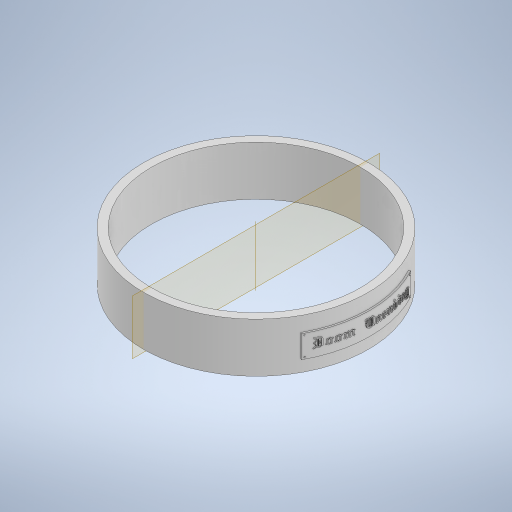
# Autodesk Inventor part: DoomUnending
Saved by Autodesk Inventor 2023 (Build 270158000, 158)
## iProperties
Created: 2023-04-08
Part Number: DoomUnending
Material: Generic
Document SubType Name: Modeling
Designer: dntpa
Density: 1 g/cm^3
Appearance: Default
Author: dntpa
## iProperties of the stored document CanisInvictoria_3DPrint.ipt
Created: 2023-04-08
Part Number: CanisInvictoria_3DPrint
Material: Generic
Document SubType Name: Modeling
Designer: dntpa
Density: 1 g/cm^3
Appearance: Default
Author: dntpa
Autodesk Inventor part; units mm, degrees
ref_plane "XZ Plane" through (0, 0, 0) normal (0, 1, 0) x (-1, 0, 0)
ref_plane "XY Plane" through (0, 0, 0) normal (0, 0, 1) x (1, 0, 0)
sketch "Sketch1" plane through (0, 0, 0) normal (0, 1, 0) x (-1, 0, 0)
  circle A0 centre (0, 0) radius 50
  circle A1 centre (0, 0) radius 46.5
  dimension "d0" = 100
  dimension "d1" = 93
  constraints: 2 centre point, 2 coincident
  measures "d0" diameter of A0
  measures "d1" diameter of A1
extrude "Extrusion1" add sketch "Sketch1" along normal blind 22
ref_plane "Work Plane1" through (60, 0, 0) normal (1, 0, 0) x (0, 1, 0)
sketch "Text" plane through (60, 0, 0) normal (1, 0, 0) x (0, 1, 0)
  line L0 (15.4535, 25) -> (15.4535, -25) construction
  line L1 (15.4535, -25) -> (5.4535, -25) construction
  line L2 (5.4535, -25) -> (5.4535, 25) construction
  line L3 (5.4535, 25) -> (15.4535, 25) construction
  line L4 (22, -50) -> (22, 50) projected
  line L5 (5.4535, 25) -> (15.4535, 25)
  line L6 (15.4535, 25) -> (15.4535, -25)
  line L7 (15.4535, -25) -> (5.4535, -25)
  line L8 (5.4535, -25) -> (5.4535, 25)
  line L9 (15.4535, 25) -> (15.4535, 0)
  line L10 (15.4535, 0) -> (15.4535, -25)
  circle A0 centre (14.7035, 24.25) radius 0.375
  line L11 (22, 0) -> (0, 0)
  line L12 (10.4535, 25) -> (10.4535, -25)
  circle A1 centre (14.7035, -24.25) radius 0.375
  circle A2 centre (6.2035, 24.25) radius 0.375
  circle A3 centre (6.2035, -24.25) radius 0.375
  line L13 (9.6365, 18.3354) -> (9.6365, 18.7286)
  line L14 (9.6365, 18.7286) -> (9.4598, 19.0748)
  line L15 (9.4598, 19.0748) -> (9.0883, 19.45)
  line L16 (9.0883, 19.45) -> (9.2758, 19.8359)
  line L17 (9.2758, 19.8359) -> (9.2758, 20.7232)
  spline S0 degree 2 poles (9.2758, 20.7232) (9.2578, 20.7881) (9.1424, 21.2606) (9.0414, 21.6754) knots 0 0 0 1 2 2 2
  line L18 (9.0414, 21.6754) -> (9.2037, 21.4265)
  line L19 (9.2037, 21.4265) -> (9.5319, 20.9288)
  line L20 (9.5319, 20.9288) -> (9.7195, 20.3733)
  line L21 (9.7195, 20.3733) -> (9.7195, 19.8647)
  line L22 (9.7195, 19.8647) -> (12.5328, 19.8647)
  line L23 (12.5328, 19.8647) -> (12.5328, 20.9179)
  spline S1 degree 2 poles (12.5328, 20.9179) (12.5689, 21.0009) (12.6627, 21.1885) (12.7204, 21.2967) knots 0 0 0 1 2 2 2
  spline S2 degree 2 poles (12.7204, 21.2967) (12.7709, 21.3472) (12.8971, 21.4734) (12.9764, 21.5491) knots 0 0 0 1 2 2 2
  line L24 (12.9764, 21.5491) -> (12.9764, 18.9089)
  line L25 (12.9764, 18.9089) -> (12.7853, 18.5266)
  line L26 (12.7853, 18.5266) -> (12.403, 18.3354)
  line L27 (12.403, 18.3354) -> (9.6365, 18.3354)
  line L28 (9.705, 18.7791) -> (10.5562, 18.7791)
  line L29 (10.5562, 18.7791) -> (10.7222, 19.1073)
  line L30 (10.7222, 19.1073) -> (10.7222, 19.45)
  line L31 (10.7222, 19.45) -> (10.5562, 19.7782)
  line L32 (10.5562, 19.7782) -> (9.7195, 19.7782)
  line L33 (9.7195, 19.7782) -> (9.7195, 19.6339)
  spline S3 degree 2 poles (9.7195, 19.6339) (9.7159, 19.6303) (9.6329, 19.3634) (9.5427, 19.1037) knots 0 0 0 1 2 2 2
  line L34 (9.5427, 19.1037) -> (9.705, 18.7791)
  spline S4 degree 2 poles (10.5743, 20.3228) (10.4949, 20.3589) (10.3074, 20.4491) (10.1956, 20.5068) knots 0 0 0 1 2 2 2
  spline S5 degree 2 poles (10.1956, 20.5068) (10.1451, 20.5573) (10.0224, 20.6871) (9.9431, 20.7665) knots 0 0 0 1 2 2 2
  line L35 (9.9431, 20.7665) -> (10.9061, 20.7665)
  line L36 (10.9061, 20.7665) -> (10.9061, 21.0694)
  line L37 (10.9061, 21.0694) -> (10.6681, 21.3111)
  line L38 (10.6681, 21.3111) -> (11.1406, 21.3111)
  line L39 (11.1406, 21.3111) -> (11.3498, 21.1055)
  line L40 (11.3498, 21.1055) -> (11.3498, 20.7665)
  line L41 (11.3498, 20.7665) -> (11.4976, 20.7665)
  spline S6 degree 2 poles (11.4976, 20.7665) (11.5806, 20.7304) (11.7645, 20.6402) (11.8764, 20.5825) knots 0 0 0 1 2 2 2
  spline S7 degree 2 poles (11.8764, 20.5825) (11.9269, 20.532) (12.0495, 20.4022) (12.1288, 20.3228) knots 0 0 0 1 2 2 2
  line L42 (12.1288, 20.3228) -> (10.5743, 20.3228)
  line L43 (11.696, 18.7791) -> (12.3777, 18.7791)
  line L44 (12.3777, 18.7791) -> (12.5328, 18.9342)
  line L45 (12.5328, 18.9342) -> (12.5328, 19.7782)
  line L46 (12.5328, 19.7782) -> (11.696, 19.7782)
  line L47 (11.696, 19.7782) -> (11.5301, 19.4463)
  line L48 (11.5301, 19.4463) -> (11.5301, 19.1073)
  line L49 (11.5301, 19.1073) -> (11.696, 18.7791)
  line L50 (10.65, 18.7791) -> (11.6022, 18.7791)
  line L51 (11.6022, 18.7791) -> (11.4471, 19.0893)
  line L52 (11.4471, 19.0893) -> (11.4471, 19.4716)
  line L53 (11.4471, 19.4716) -> (11.6022, 19.7782)
  line L54 (11.6022, 19.7782) -> (10.65, 19.7782)
  line L55 (10.65, 19.7782) -> (10.8051, 19.4716)
  line L56 (10.8051, 19.4716) -> (10.8051, 19.0893)
  line L57 (10.8051, 19.0893) -> (10.65, 18.7791)
  line L58 (11.3498, 14.5518) -> (11.1045, 15.046)
  line L59 (11.1045, 15.046) -> (9.4562, 15.046)
  line L60 (9.4562, 15.046) -> (9.4562, 15.4463)
  spline S8 degree 2 poles (9.4562, 15.4463) (9.4526, 15.4608) (9.4273, 15.5473) (9.4021, 15.6231) knots 0 0 0 1 2 2 2
  line L61 (9.4021, 15.6231) -> (9.283, 15.9766)
  spline S9 degree 2 poles (9.283, 15.9766) (9.247, 16.0415) (9.1532, 16.2363) (9.0883, 16.3661) knots 0 0 0 1 2 2 2
  line L62 (9.0883, 16.3661) -> (9.283, 16.5609)
  spline S10 degree 2 poles (9.283, 16.5609) (9.3443, 16.6943) (9.4562, 16.9107) knots 0 0 0 1 1 1
  line L63 (9.4562, 16.9107) -> (9.4562, 17.4373)
  line L64 (9.4562, 17.4373) -> (9.705, 16.9396)
  line L65 (9.705, 16.9396) -> (11.3498, 16.9396)
  line L66 (11.3498, 16.9396) -> (11.3498, 16.5392)
  spline S11 degree 2 poles (11.3498, 16.5392) (11.357, 16.5284) (11.3822, 16.4382) (11.4075, 16.3661) knots 0 0 0 1 2 2 2
  line L67 (11.4075, 16.3661) -> (11.5265, 16.009)
  spline S12 degree 2 poles (11.5265, 16.009) (11.559, 15.9405) (11.6563, 15.7493) (11.7213, 15.6231) knots 0 0 0 1 2 2 2
  spline S13 degree 2 poles (11.7213, 15.6231) (11.6744, 15.5726) (11.577, 15.4752) (11.5265, 15.4247) knots 0 0 0 1 2 2 2
  spline S14 degree 2 poles (11.5265, 15.4247) (11.5193, 15.4139) (11.4327, 15.2444) (11.3498, 15.0785) knots 0 0 0 1 2 2 2
  line L68 (11.3498, 15.0785) -> (11.3498, 14.5518)
  line L69 (9.5283, 15.4896) -> (11.1009, 15.4896)
  spline S15 degree 2 poles (11.1009, 15.4896) (11.1297, 15.5582) (11.2163, 15.7313) (11.2704, 15.8395) knots 0 0 0 1 2 2 2
  spline S16 degree 2 poles (11.2704, 15.8395) (11.3101, 15.8756) (11.393, 15.9585) (11.4435, 16.0018) knots 0 0 0 1 2 2 2
  line L70 (11.4435, 16.0018) -> (11.2776, 16.4959)
  line L71 (11.2776, 16.4959) -> (9.705, 16.4959)
  spline S17 degree 2 poles (9.705, 16.4959) (9.6762, 16.431) (9.5896, 16.2543) (9.5355, 16.1497) knots 0 0 0 1 2 2 2
  line L72 (9.5355, 16.1497) -> (9.3624, 15.9838)
  line L73 (9.3624, 15.9838) -> (9.5283, 15.4896)
  line L74 (11.3498, 11.2624) -> (11.1045, 11.7565)
  line L75 (11.1045, 11.7565) -> (9.4562, 11.7565)
  line L76 (9.4562, 11.7565) -> (9.4562, 12.1569)
  spline S18 degree 2 poles (9.4562, 12.1569) (9.4526, 12.1713) (9.4273, 12.2579) (9.4021, 12.3336) knots 0 0 0 1 2 2 2
  line L77 (9.4021, 12.3336) -> (9.283, 12.6871)
  spline S19 degree 2 poles (9.283, 12.6871) (9.247, 12.752) (9.1532, 12.9468) (9.0883, 13.0766) knots 0 0 0 1 2 2 2
  line L78 (9.0883, 13.0766) -> (9.283, 13.2714)
  spline S20 degree 2 poles (9.283, 13.2714) (9.3443, 13.4049) (9.4562, 13.6213) knots 0 0 0 1 1 1
  line L79 (9.4562, 13.6213) -> (9.4562, 14.1479)
  line L80 (9.4562, 14.1479) -> (9.705, 13.6501)
  line L81 (9.705, 13.6501) -> (11.3498, 13.6501)
  line L82 (11.3498, 13.6501) -> (11.3498, 13.2498)
  spline S21 degree 2 poles (11.3498, 13.2498) (11.357, 13.239) (11.3822, 13.1488) (11.4075, 13.0766) knots 0 0 0 1 2 2 2
  line L83 (11.4075, 13.0766) -> (11.5265, 12.7196)
  spline S22 degree 2 poles (11.5265, 12.7196) (11.559, 12.651) (11.6563, 12.4599) (11.7213, 12.3336) knots 0 0 0 1 2 2 2
  spline S23 degree 2 poles (11.7213, 12.3336) (11.6744, 12.2831) (11.577, 12.1858) (11.5265, 12.1353) knots 0 0 0 1 2 2 2
  spline S24 degree 2 poles (11.5265, 12.1353) (11.5193, 12.1244) (11.4327, 11.9549) (11.3498, 11.789) knots 0 0 0 1 2 2 2
  line L84 (11.3498, 11.789) -> (11.3498, 11.2624)
  line L85 (9.5283, 12.2002) -> (11.1009, 12.2002)
  spline S25 degree 2 poles (11.1009, 12.2002) (11.1297, 12.2687) (11.2163, 12.4418) (11.2704, 12.55) knots 0 0 0 1 2 2 2
  spline S26 degree 2 poles (11.2704, 12.55) (11.3101, 12.5861) (11.393, 12.6691) (11.4435, 12.7124) knots 0 0 0 1 2 2 2
  line L86 (11.4435, 12.7124) -> (11.2776, 13.2065)
  line L87 (11.2776, 13.2065) -> (9.705, 13.2065)
  spline S27 degree 2 poles (9.705, 13.2065) (9.6762, 13.1416) (9.5896, 12.9648) (9.5355, 12.8602) knots 0 0 0 1 2 2 2
  line L88 (9.5355, 12.8602) -> (9.3624, 12.6943)
  line L89 (9.3624, 12.6943) -> (9.5283, 12.2002)
  line L90 (11.3498, 6.523) -> (11.1009, 7.0207)
  line L91 (11.1009, 7.0207) -> (9.6942, 7.0207)
  line L92 (9.6942, 7.0207) -> (9.5391, 6.8656)
  line L93 (9.5391, 6.8656) -> (9.5391, 6.6023)
  line L94 (9.5391, 6.6023) -> (9.081, 7.0604)
  line L95 (9.081, 7.0604) -> (9.4814, 7.4644)
  line L96 (9.4814, 7.4644) -> (11.1009, 7.4644)
  line L97 (11.1009, 7.4644) -> (11.2632, 7.7962)
  line L98 (11.2632, 7.7962) -> (11.2632, 7.9621)
  line L99 (11.2632, 7.9621) -> (11.0937, 8.4671)
  line L100 (11.0937, 8.4671) -> (9.705, 8.4671)
  line L101 (9.705, 8.4671) -> (9.5067, 8.0775)
  line L102 (9.5067, 8.0775) -> (9.081, 8.5104)
  spline S28 degree 2 poles (9.081, 8.5104) (9.2686, 8.7015) (9.2794, 8.716) knots 0 0 0 1 1 1
  spline S29 degree 2 poles (9.2794, 8.716) (9.2866, 8.7304) (9.3912, 8.9324) (9.4886, 9.1235) knots 0 0 0 1 2 2 2
  line L103 (9.4886, 9.1235) -> (9.6942, 8.9107)
  line L104 (9.6942, 8.9107) -> (11.1009, 8.9107)
  line L105 (11.1009, 8.9107) -> (11.2632, 9.2462)
  line L106 (11.2632, 9.2462) -> (11.2632, 9.4085)
  spline S30 degree 2 poles (11.2632, 9.4085) (11.2632, 9.4698) (11.0937, 9.917) knots 0 0 0 1 1 1
  line L107 (11.0937, 9.917) -> (9.705, 9.917)
  line L108 (9.705, 9.917) -> (9.5067, 9.5239)
  line L109 (9.5067, 9.5239) -> (9.081, 9.9567)
  spline S31 degree 2 poles (9.081, 9.9567) (9.2614, 10.1407) (9.2975, 10.1984) knots 0 0 0 1 1 1
  spline S32 degree 2 poles (9.2975, 10.1984) (9.3011, 10.202) (9.3768, 10.3571) (9.4562, 10.5086) knots 0 0 0 1 2 2 2
  line L110 (9.4562, 10.5086) -> (9.4562, 10.8584)
  line L111 (9.4562, 10.8584) -> (9.705, 10.3607)
  line L112 (9.705, 10.3607) -> (11.1117, 10.3607)
  line L113 (11.1117, 10.3607) -> (11.2668, 10.5158)
  line L114 (11.2668, 10.5158) -> (11.2668, 10.7791)
  line L115 (11.2668, 10.7791) -> (11.7249, 10.321)
  line L116 (11.7249, 10.321) -> (11.3245, 9.917)
  line L117 (11.3245, 9.917) -> (11.1874, 9.917)
  spline S33 degree 2 poles (11.1874, 9.917) (11.2127, 9.8449) (11.2668, 9.6862) (11.2957, 9.5924) knots 0 0 0 1 2 2 2
  spline S34 degree 2 poles (11.2957, 9.5924) (11.3065, 9.5455) (11.3498, 9.4301) knots 0 0 0 1 1 1
  spline S35 degree 2 poles (11.3498, 9.4301) (11.3678, 9.3832) (11.4544, 9.2101) (11.5265, 9.0766) knots 0 0 0 1 2 2 2
  spline S36 degree 2 poles (11.5265, 9.0766) (11.5409, 9.055) (11.7249, 8.8711) knots 0 0 0 1 1 1
  line L118 (11.7249, 8.8711) -> (11.3245, 8.4671)
  line L119 (11.3245, 8.4671) -> (11.1802, 8.4671)
  spline S37 degree 2 poles (11.1802, 8.4671) (11.2019, 8.3986) (11.2848, 8.1569) (11.3425, 7.9838) knots 0 0 0 1 2 2 2
  spline S38 degree 2 poles (11.3425, 7.9838) (11.4111, 7.7998) (11.5265, 7.6303) knots 0 0 0 1 1 1
  spline S39 degree 2 poles (11.5265, 7.6303) (11.5409, 7.6087) (11.7249, 7.4247) knots 0 0 0 1 1 1
  spline S40 degree 2 poles (11.7249, 7.4247) (11.5445, 7.2444) (11.5049, 7.1794) knots 0 0 0 1 1 1
  spline S41 degree 2 poles (11.5049, 7.1794) (11.4868, 7.1578) (11.3498, 6.8729) knots 0 0 0 1 1 1
  line L120 (11.3498, 6.8729) -> (11.3498, 6.523)
  line L121 (9.5391, -1.6032) -> (9.081, -1.1416)
  line L122 (9.081, -1.1416) -> (9.4453, -0.7701)
  spline S42 degree 2 poles (9.4453, -0.7701) (9.384, -0.6582) (9.283, -0.4346) knots 0 0 0 1 1 1
  spline S43 degree 2 poles (9.283, -0.4346) (9.2758, -0.4166) (9.2253, -0.2723) (9.182, -0.1461) knots 0 0 0 1 2 2 2
  line L123 (9.182, -0.1461) -> (9.0955, 0.1172)
  line L124 (9.0955, 0.1172) -> (9.0955, 0.6727)
  spline S44 degree 2 poles (9.0955, 0.6727) (9.1388, 0.8025) (9.2325, 1.0803) (9.283, 1.2317) knots 0 0 0 1 2 2 2
  line L125 (9.283, 1.2317) -> (9.4057, 1.3544)
  line L126 (9.4057, 1.3544) -> (9.6509, 1.6069)
  spline S45 degree 2 poles (9.6509, 1.6069) (9.6617, 1.6141) (9.7772, 1.6682) knots 0 0 0 1 1 1
  line L127 (9.7772, 1.6682) -> (10.026, 1.7872)
  line L128 (10.026, 1.7872) -> (10.3939, 1.9134)
  spline S46 degree 2 poles (10.3939, 1.9134) (10.4012, 1.917) (10.448, 1.9351) (10.4841, 1.9531) knots 0 0 0 1 2 2 2
  spline S47 degree 2 poles (10.4841, 1.9531) (10.531, 1.9748) (10.5779, 1.9748) knots 0 0 0 1 1 1
  line L129 (10.5779, 1.9748) -> (11.3137, 1.9748)
  spline S48 degree 2 poles (11.3137, 1.9748) (11.357, 1.9748) (11.4075, 1.9531) knots 0 0 0 1 1 1
  spline S49 degree 2 poles (11.4075, 1.9531) (11.4435, 1.9351) (11.4868, 1.9134) (11.4976, 1.9134) knots 0 0 0 1 2 2 2
  line L130 (11.4976, 1.9134) -> (11.8655, 1.7908)
  spline S50 degree 2 poles (11.8655, 1.7908) (11.8872, 1.78) (12.0026, 1.7223) (12.1, 1.6754) knots 0 0 0 1 2 2 2
  line L131 (12.1, 1.6754) -> (12.5689, 1.4445)
  line L132 (12.5689, 1.4445) -> (11.4832, 1.7115)
  line L133 (11.4832, 1.7115) -> (10.9494, 1.7115)
  spline S51 degree 2 poles (10.9494, 1.7115) (10.9386, 1.7078) (10.8484, 1.6826) (10.7763, 1.6573) knots 0 0 0 1 2 2 2
  line L134 (10.7763, 1.6573) -> (10.4156, 1.5383)
  line L135 (10.4156, 1.5383) -> (10.1847, 1.4157)
  spline S52 degree 2 poles (10.1847, 1.4157) (10.1415, 1.3977) (10.0657, 1.3544) knots 0 0 0 1 1 1
  line L136 (10.0657, 1.3544) -> (9.8349, 1.1235)
  line L137 (9.8349, 1.1235) -> (9.7159, 1.0081)
  line L138 (9.7159, 1.0081) -> (9.5391, 0.4815)
  line L139 (9.5391, 0.4815) -> (9.5391, -0.1966)
  line L140 (9.5391, -0.1966) -> (12.3416, -0.1966)
  line L141 (12.3416, -0.1966) -> (12.2118, 0.3156)
  line L142 (12.2118, 0.3156) -> (12.2118, 0.2651)
  line L143 (12.2118, 0.2651) -> (10.5743, 0.2651)
  spline S53 degree 2 poles (10.5743, 0.2651) (10.4913, 0.3012) (10.3074, 0.3913) (10.1956, 0.4491) knots 0 0 0 1 2 2 2
  spline S54 degree 2 poles (10.1956, 0.4491) (10.1451, 0.4996) (10.0224, 0.6294) (9.9431, 0.7087) knots 0 0 0 1 2 2 2
  line L144 (9.9431, 0.7087) -> (11.8619, 0.7087)
  line L145 (11.8619, 0.7087) -> (12.2479, 0.5176)
  line L146 (12.2479, 0.5176) -> (12.3705, 0.0198)
  spline S55 degree 2 poles (12.3705, 0.0198) (12.3777, -0.0126) (12.4102, -0.1353) (12.4354, -0.2218) knots 0 0 0 1 2 2 2
  line L147 (12.4354, -0.2218) -> (12.6122, -0.5753)
  line L148 (12.6122, -0.5753) -> (12.9909, -0.9612)
  spline S56 degree 2 poles (12.9909, -0.9612) (12.8214, -1.1344) (12.7528, -1.2498) knots 0 0 0 1 1 1
  spline S57 degree 2 poles (12.7528, -1.2498) (12.742, -1.2606) (12.6518, -1.4337) (12.5725, -1.5996) knots 0 0 0 1 2 2 2
  line L149 (12.5725, -1.5996) -> (12.3669, -1.1849)
  line L150 (12.3669, -1.1849) -> (9.8709, -1.1849)
  line L151 (9.8709, -1.1849) -> (9.5391, -1.3472)
  line L152 (9.5391, -1.3472) -> (9.5391, -1.6032)
  line L153 (9.7086, -0.7412) -> (10.7222, -0.7412)
  line L154 (10.7222, -0.7412) -> (10.7222, -0.2795)
  line L155 (10.7222, -0.2795) -> (9.5535, -0.2795)
  line L156 (9.5535, -0.2795) -> (9.7086, -0.7412)
  line L157 (13.0847, 0.2759) -> (12.5328, 0.835)
  line L158 (12.5328, 0.835) -> (12.5328, 1.2173)
  line L159 (12.5328, 1.2173) -> (12.7095, 1.7475)
  line L160 (12.7095, 1.7475) -> (12.4246, 2.3282)
  line L161 (12.4246, 2.3282) -> (12.9764, 1.7692)
  line L162 (12.9764, 1.7692) -> (12.9764, 1.3868)
  spline S58 degree 2 poles (12.9764, 1.3868) (12.9548, 1.3147) (12.8646, 1.0514) (12.7997, 0.853) knots 0 0 0 1 2 2 2
  line L163 (12.7997, 0.853) -> (13.0847, 0.2759)
  line L164 (11.5301, -0.7412) -> (12.3741, -0.7412)
  line L165 (12.3741, -0.7412) -> (12.522, -0.5897)
  line L166 (12.522, -0.5897) -> (12.3669, -0.2759)
  line L167 (12.3669, -0.2759) -> (11.5301, -0.2759)
  line L168 (11.5301, -0.2759) -> (11.5301, -0.7412)
  line L169 (10.8051, -0.7412) -> (11.4471, -0.7412)
  line L170 (11.4471, -0.7412) -> (11.4471, -0.2759)
  line L171 (11.4471, -0.2759) -> (10.8051, -0.2759)
  line L172 (10.8051, -0.2759) -> (10.8051, -0.7412)
  line L173 (11.3498, -4.9684) -> (11.1009, -4.4743)
  line L174 (11.1009, -4.4743) -> (9.6942, -4.4743)
  line L175 (9.6942, -4.4743) -> (9.5391, -4.6294)
  line L176 (9.5391, -4.6294) -> (9.5391, -4.8927)
  line L177 (9.5391, -4.8927) -> (9.081, -4.431)
  line L178 (9.081, -4.431) -> (9.4814, -4.0307)
  line L179 (9.4814, -4.0307) -> (11.1009, -4.0307)
  line L180 (11.1009, -4.0307) -> (11.2632, -3.6952)
  line L181 (11.2632, -3.6952) -> (11.2632, -3.5329)
  line L182 (11.2632, -3.5329) -> (11.0937, -3.0243)
  line L183 (11.0937, -3.0243) -> (9.705, -3.0243)
  line L184 (9.705, -3.0243) -> (9.5067, -3.4175)
  line L185 (9.5067, -3.4175) -> (9.081, -2.9847)
  spline S59 degree 2 poles (9.081, -2.9847) (9.2614, -2.8007) (9.2975, -2.743) knots 0 0 0 1 1 1
  spline S60 degree 2 poles (9.2975, -2.743) (9.3011, -2.7394) (9.3768, -2.5843) (9.4562, -2.4328) knots 0 0 0 1 2 2 2
  line L186 (9.4562, -2.4328) -> (9.4562, -2.083)
  line L187 (9.4562, -2.083) -> (9.705, -2.5807)
  line L188 (9.705, -2.5807) -> (11.1117, -2.5807)
  line L189 (11.1117, -2.5807) -> (11.2668, -2.4256)
  line L190 (11.2668, -2.4256) -> (11.2668, -2.1623)
  line L191 (11.2668, -2.1623) -> (11.7249, -2.6204)
  line L192 (11.7249, -2.6204) -> (11.3245, -3.0243)
  line L193 (11.3245, -3.0243) -> (11.1802, -3.0243)
  spline S61 degree 2 poles (11.1802, -3.0243) (11.2019, -3.1109) (11.2848, -3.3526) (11.3425, -3.5113) knots 0 0 0 1 2 2 2
  line L194 (11.3425, -3.5113) -> (11.4616, -3.7457)
  spline S62 degree 2 poles (11.4616, -3.7457) (11.476, -3.7782) (11.5265, -3.8647) knots 0 0 0 1 1 1
  spline S63 degree 2 poles (11.5265, -3.8647) (11.5373, -3.8792) (11.7249, -4.0703) knots 0 0 0 1 1 1
  spline S64 degree 2 poles (11.7249, -4.0703) (11.5445, -4.2507) (11.5049, -4.3156) knots 0 0 0 1 1 1
  spline S65 degree 2 poles (11.5049, -4.3156) (11.4868, -4.3336) (11.3498, -4.6222) knots 0 0 0 1 1 1
  line L195 (11.3498, -4.6222) -> (11.3498, -4.9684)
  line L196 (10.935, -7.6014) -> (10.1956, -6.3138)
  line L197 (10.1956, -6.3138) -> (9.705, -6.3138)
  line L198 (9.705, -6.3138) -> (9.5391, -6.6456)
  line L199 (9.5391, -6.6456) -> (9.5391, -6.9919)
  line L200 (9.5391, -6.9919) -> (9.3696, -6.6492)
  spline S66 degree 2 poles (9.3696, -6.6492) (9.348, -6.6132) (9.3047, -6.5266) (9.2794, -6.4797) knots 0 0 0 1 2 2 2
  spline S67 degree 2 poles (9.2794, -6.4797) (9.2686, -6.4653) (9.081, -6.2741) knots 0 0 0 1 1 1
  spline S68 degree 2 poles (9.081, -6.2741) (9.2614, -6.0902) (9.2975, -6.0325) knots 0 0 0 1 1 1
  spline S69 degree 2 poles (9.2975, -6.0325) (9.3011, -6.0289) (9.3768, -5.8738) (9.4562, -5.7223) knots 0 0 0 1 2 2 2
  line L201 (9.4562, -5.7223) -> (9.4562, -5.3724)
  line L202 (9.4562, -5.3724) -> (9.705, -5.8702)
  line L203 (9.705, -5.8702) -> (11.3389, -5.8702)
  line L204 (11.3389, -5.8702) -> (11.5301, -6.6204)
  spline S70 degree 2 poles (11.5301, -6.6204) (11.5373, -6.642) (11.7213, -7.0063) knots 0 0 0 1 1 1
  line L205 (11.7213, -7.0063) -> (10.935, -7.6014)
  line L206 (10.7582, -7.1326) -> (11.4363, -6.624)
  line L207 (11.4363, -6.624) -> (11.2812, -6.3138)
  line L208 (11.2812, -6.3138) -> (10.2929, -6.3138)
  line L209 (10.2929, -6.3138) -> (10.7582, -7.1326)
  line L210 (11.3498, -10.8224) -> (11.1009, -10.3282)
  line L211 (11.1009, -10.3282) -> (9.6942, -10.3282)
  line L212 (9.6942, -10.3282) -> (9.5391, -10.4833)
  line L213 (9.5391, -10.4833) -> (9.5391, -10.7466)
  line L214 (9.5391, -10.7466) -> (9.081, -10.2849)
  line L215 (9.081, -10.2849) -> (9.4814, -9.8846)
  line L216 (9.4814, -9.8846) -> (11.1009, -9.8846)
  line L217 (11.1009, -9.8846) -> (11.2632, -9.5491)
  line L218 (11.2632, -9.5491) -> (11.2632, -9.3868)
  line L219 (11.2632, -9.3868) -> (11.0937, -8.8783)
  line L220 (11.0937, -8.8783) -> (9.705, -8.8783)
  line L221 (9.705, -8.8783) -> (9.5067, -9.2714)
  line L222 (9.5067, -9.2714) -> (9.081, -8.8386)
  spline S71 degree 2 poles (9.081, -8.8386) (9.2614, -8.6546) (9.2975, -8.5969) knots 0 0 0 1 1 1
  spline S72 degree 2 poles (9.2975, -8.5969) (9.3011, -8.5933) (9.3768, -8.4382) (9.4562, -8.2867) knots 0 0 0 1 2 2 2
  line L223 (9.4562, -8.2867) -> (9.4562, -7.9369)
  line L224 (9.4562, -7.9369) -> (9.705, -8.4346)
  line L225 (9.705, -8.4346) -> (11.1117, -8.4346)
  line L226 (11.1117, -8.4346) -> (11.2668, -8.2795)
  line L227 (11.2668, -8.2795) -> (11.2668, -8.0162)
  line L228 (11.2668, -8.0162) -> (11.7249, -8.4743)
  line L229 (11.7249, -8.4743) -> (11.3245, -8.8783)
  line L230 (11.3245, -8.8783) -> (11.1802, -8.8783)
  spline S73 degree 2 poles (11.1802, -8.8783) (11.2019, -8.9648) (11.2848, -9.2065) (11.3425, -9.3652) knots 0 0 0 1 2 2 2
  line L231 (11.3425, -9.3652) -> (11.4616, -9.5996)
  spline S74 degree 2 poles (11.4616, -9.5996) (11.476, -9.6321) (11.5265, -9.7187) knots 0 0 0 1 1 1
  spline S75 degree 2 poles (11.5265, -9.7187) (11.5373, -9.7331) (11.7249, -9.9243) knots 0 0 0 1 1 1
  spline S76 degree 2 poles (11.7249, -9.9243) (11.5445, -10.1046) (11.5049, -10.1695) knots 0 0 0 1 1 1
  spline S77 degree 2 poles (11.5049, -10.1695) (11.4868, -10.1876) (11.3498, -10.4761) knots 0 0 0 1 1 1
  line L232 (11.3498, -10.4761) -> (11.3498, -10.8224)
  line L233 (9.4562, -13.6177) -> (9.4562, -13.2173)
  spline S78 degree 2 poles (9.4562, -13.2173) (9.4526, -13.2029) (9.4273, -13.1163) (9.4021, -13.0406) knots 0 0 0 1 2 2 2
  line L234 (9.4021, -13.0406) -> (9.283, -12.6871)
  spline S79 degree 2 poles (9.283, -12.6871) (9.247, -12.6222) (9.1532, -12.4274) (9.0883, -12.2976) knots 0 0 0 1 2 2 2
  line L235 (9.0883, -12.2976) -> (9.283, -12.1028)
  spline S80 degree 2 poles (9.283, -12.1028) (9.3443, -11.9693) (9.4562, -11.7529) knots 0 0 0 1 1 1
  line L236 (9.4562, -11.7529) -> (9.4562, -11.2263)
  line L237 (9.4562, -11.2263) -> (9.705, -11.7241)
  line L238 (9.705, -11.7241) -> (11.3389, -11.7241)
  line L239 (11.3389, -11.7241) -> (11.4003, -11.9152)
  line L240 (11.4003, -11.9152) -> (11.5265, -12.294)
  line L241 (11.5265, -12.294) -> (11.6816, -12.5969)
  line L242 (11.6816, -12.5969) -> (12.5797, -11.6988)
  line L243 (12.5797, -11.6988) -> (12.9981, -12.33)
  line L244 (12.9981, -12.33) -> (12.4138, -12.5284)
  line L245 (12.4138, -12.5284) -> (11.3245, -13.6177)
  line L246 (11.3245, -13.6177) -> (9.4562, -13.6177)
  line L247 (9.5283, -13.174) -> (11.1117, -13.174)
  line L248 (11.1117, -13.174) -> (11.6167, -12.6655)
  line L249 (11.6167, -12.6655) -> (11.2848, -12.1677)
  line L250 (11.2848, -12.1677) -> (9.705, -12.1677)
  spline S81 degree 2 poles (9.705, -12.1677) (9.6762, -12.2326) (9.5896, -12.4094) (9.5355, -12.514) knots 0 0 0 1 2 2 2
  line L251 (9.5355, -12.514) -> (9.3624, -12.6799)
  line L252 (9.3624, -12.6799) -> (9.5283, -13.174)
  line L253 (9.5391, -15.6916) -> (9.081, -15.2335)
  line L254 (9.081, -15.2335) -> (9.4814, -14.8296)
  line L255 (9.4814, -14.8296) -> (11.1009, -14.8296)
  line L256 (11.1009, -14.8296) -> (11.3065, -14.4148)
  spline S82 degree 2 poles (11.3065, -14.4148) (11.3498, -14.505) (11.458, -14.7178) (11.5229, -14.844) knots 0 0 0 1 2 2 2
  spline S83 degree 2 poles (11.5229, -14.844) (11.5409, -14.8656) (11.7249, -15.0532) knots 0 0 0 1 1 1
  spline S84 degree 2 poles (11.7249, -15.0532) (11.5409, -15.2371) (11.5229, -15.2588) knots 0 0 0 1 1 1
  spline S85 degree 2 poles (11.5229, -15.2588) (11.5193, -15.266) (11.4147, -15.4788) (11.3065, -15.688) knots 0 0 0 1 2 2 2
  line L257 (11.3065, -15.688) -> (11.1009, -15.2732)
  line L258 (11.1009, -15.2732) -> (9.6942, -15.2732)
  line L259 (9.6942, -15.2732) -> (9.5391, -15.4283)
  line L260 (9.5391, -15.4283) -> (9.5391, -15.6916)
  line L261 (12.5617, -15.486) -> (12.3452, -15.0496)
  line L262 (12.3452, -15.0496) -> (12.5617, -14.6168)
  line L263 (12.5617, -14.6168) -> (12.9909, -15.0496)
  line L264 (12.9909, -15.0496) -> (12.5617, -15.486)
  line L265 (11.3498, -19.0604) -> (11.1009, -18.5663)
  line L266 (11.1009, -18.5663) -> (9.6942, -18.5663)
  line L267 (9.6942, -18.5663) -> (9.5391, -18.7214)
  line L268 (9.5391, -18.7214) -> (9.5391, -18.9847)
  line L269 (9.5391, -18.9847) -> (9.081, -18.523)
  line L270 (9.081, -18.523) -> (9.4814, -18.1226)
  line L271 (9.4814, -18.1226) -> (11.1009, -18.1226)
  line L272 (11.1009, -18.1226) -> (11.2632, -17.7872)
  line L273 (11.2632, -17.7872) -> (11.2632, -17.6249)
  line L274 (11.2632, -17.6249) -> (11.0937, -17.1163)
  line L275 (11.0937, -17.1163) -> (9.705, -17.1163)
  line L276 (9.705, -17.1163) -> (9.5067, -17.5095)
  line L277 (9.5067, -17.5095) -> (9.081, -17.0766)
  spline S86 degree 2 poles (9.081, -17.0766) (9.2614, -16.8927) (9.2975, -16.835) knots 0 0 0 1 1 1
  spline S87 degree 2 poles (9.2975, -16.835) (9.3011, -16.8314) (9.3768, -16.6763) (9.4562, -16.5248) knots 0 0 0 1 2 2 2
  line L278 (9.4562, -16.5248) -> (9.4562, -16.1749)
  line L279 (9.4562, -16.1749) -> (9.705, -16.6727)
  line L280 (9.705, -16.6727) -> (11.1117, -16.6727)
  line L281 (11.1117, -16.6727) -> (11.2668, -16.5176)
  line L282 (11.2668, -16.5176) -> (11.2668, -16.2543)
  line L283 (11.2668, -16.2543) -> (11.7249, -16.7124)
  line L284 (11.7249, -16.7124) -> (11.3245, -17.1163)
  line L285 (11.3245, -17.1163) -> (11.1802, -17.1163)
  spline S88 degree 2 poles (11.1802, -17.1163) (11.2019, -17.2029) (11.2848, -17.4445) (11.3425, -17.6032) knots 0 0 0 1 2 2 2
  line L286 (11.3425, -17.6032) -> (11.4616, -17.8377)
  spline S89 degree 2 poles (11.4616, -17.8377) (11.476, -17.8702) (11.5265, -17.9567) knots 0 0 0 1 1 1
  spline S90 degree 2 poles (11.5265, -17.9567) (11.5373, -17.9711) (11.7249, -18.1623) knots 0 0 0 1 1 1
  spline S91 degree 2 poles (11.7249, -18.1623) (11.5445, -18.3427) (11.5049, -18.4076) knots 0 0 0 1 1 1
  spline S92 degree 2 poles (11.5049, -18.4076) (11.4868, -18.4256) (11.3498, -18.7142) knots 0 0 0 1 1 1
  line L287 (11.3498, -18.7142) -> (11.3498, -19.0604)
  line L288 (11.3498, -22.3499) -> (11.1045, -21.8557)
  line L289 (11.1045, -21.8557) -> (8.9548, -21.8557)
  spline S93 degree 2 poles (8.9548, -21.8557) (8.825, -21.8124) (8.5581, -21.7259) (8.4138, -21.6754) knots 0 0 0 1 2 2 2
  line L290 (8.4138, -21.6754) -> (8.403, -21.6754)
  spline S94 degree 2 poles (8.403, -21.6754) (8.3164, -21.5924) (8.1288, -21.4085) (8.0206, -21.2967) knots 0 0 0 1 2 2 2
  spline S95 degree 2 poles (8.0206, -21.2967) (7.9773, -21.2065) (7.8764, -21.0117) (7.8223, -20.8999) knots 0 0 0 1 2 2 2
  line L291 (7.8223, -20.8999) -> (8.0206, -20.7015)
  spline S96 degree 2 poles (8.0206, -20.7015) (8.0278, -20.6943) (8.1144, -20.5212) (8.1974, -20.3589) knots 0 0 0 1 2 2 2
  line L292 (8.1974, -20.3589) -> (8.1974, -19.8287)
  line L293 (8.1974, -19.8287) -> (8.4571, -20.3589)
  line L294 (8.4571, -20.3589) -> (8.4571, -20.7376)
  spline S97 degree 2 poles (8.4571, -20.7376) (8.4246, -20.8097) (8.3308, -21.0009) (8.2731, -21.1163) knots 0 0 0 1 2 2 2
  line L295 (8.2731, -21.1163) -> (8.1108, -21.2714)
  line L296 (8.1108, -21.2714) -> (8.4318, -21.5924)
  line L297 (8.4318, -21.5924) -> (8.7745, -21.5924)
  spline S98 degree 2 poles (8.7745, -21.5924) (8.8177, -21.5924) (8.8682, -21.5672) knots 0 0 0 1 1 1
  spline S99 degree 2 poles (8.8682, -21.5672) (8.9368, -21.5347) (8.9548, -21.5311) knots 0 0 0 1 1 1
  line L298 (8.9548, -21.5311) -> (9.3155, -21.4121)
  line L299 (9.3155, -21.4121) -> (9.6509, -21.4121)
  spline S100 degree 2 poles (9.6509, -21.4121) (9.586, -21.2281) (9.4634, -20.9288) (9.4021, -20.8061) knots 0 0 0 1 2 2 2
  line L300 (9.4021, -20.8061) -> (9.283, -20.5717)
  spline S101 degree 2 poles (9.283, -20.5717) (9.2722, -20.5573) (9.0847, -20.3661) knots 0 0 0 1 1 1
  spline S102 degree 2 poles (9.0847, -20.3661) (9.265, -20.1821) (9.3011, -20.1244) knots 0 0 0 1 1 1
  spline S103 degree 2 poles (9.3011, -20.1244) (9.3047, -20.1208) (9.3804, -19.9657) (9.4562, -19.8142) knots 0 0 0 1 2 2 2
  line L301 (9.4562, -19.8142) -> (9.4562, -19.4644)
  line L302 (9.4562, -19.4644) -> (9.7086, -19.9621)
  line L303 (9.7086, -19.9621) -> (11.3498, -19.9621)
  line L304 (11.3498, -19.9621) -> (11.3498, -20.3625)
  spline S104 degree 2 poles (11.3498, -20.3625) (11.357, -20.3733) (11.3822, -20.4635) (11.4075, -20.5356) knots 0 0 0 1 2 2 2
  line L305 (11.4075, -20.5356) -> (11.5265, -20.8927)
  spline S105 degree 2 poles (11.5265, -20.8927) (11.559, -20.9612) (11.6563, -21.1524) (11.7213, -21.2786) knots 0 0 0 1 2 2 2
  spline S106 degree 2 poles (11.7213, -21.2786) (11.6744, -21.3291) (11.577, -21.4265) (11.5265, -21.477) knots 0 0 0 1 2 2 2
  spline S107 degree 2 poles (11.5265, -21.477) (11.5193, -21.4878) (11.4327, -21.6573) (11.3498, -21.8233) knots 0 0 0 1 2 2 2
  line L306 (11.3498, -21.8233) -> (11.3498, -22.3499)
  line L307 (9.7375, -21.4121) -> (11.1009, -21.4121)
  spline S108 degree 2 poles (11.1009, -21.4121) (11.1297, -21.3436) (11.2163, -21.1704) (11.2704, -21.0622) knots 0 0 0 1 2 2 2
  spline S109 degree 2 poles (11.2704, -21.0622) (11.3101, -21.0261) (11.393, -20.9432) (11.4435, -20.8999) knots 0 0 0 1 2 2 2
  line L308 (11.4435, -20.8999) -> (11.2776, -20.4058)
  line L309 (11.2776, -20.4058) -> (9.705, -20.4058)
  line L310 (9.705, -20.4058) -> (9.5391, -20.7376)
  line L311 (9.5391, -20.7376) -> (9.5391, -20.9035)
  line L312 (9.5391, -20.9035) -> (9.7375, -21.4121)
  dimension "d6" = 11.5465
  dimension "d10" = 0
  dimension "d11" = 10
  dimension "d12" = 50
  dimension "d25" = 0.75
  dimension "d26" = 0.75
  dimension "d27" = 0.75
  constraints: 16 end point, 5 midpoint, 4 centre point, 3 symmetric about line, 2 collinear, 2 horizontal, 2 parallel, 1 perpendicular, 5 other
  measures "d6" distance from line of L4 L12.start
  measures "d10" vertical distance of L11.start point (15.453, 0)
  measures "d11" distance between parallel lines of L0 L2
  measures "d12" distance between parallel lines of L3 L1
  measures "d25" diameter of A0
  measures "d26" distance from line of L0 A0.centre
  measures "d27" distance from line of L3 A0.centre
sketch "NamePlate" plane through (60, 0, 0) normal (1, 0, 0) x (0, 1, 0)
  line L0 (15.4535, 25) -> (5.4535, 25)
  line L1 (5.4535, 25) -> (5.4535, -25)
  line L2 (5.4535, -25) -> (15.4535, -25)
  line L3 (15.4535, -25) -> (15.4535, 25)
  point P0 (0, 0)
  point P1 (15.4535, 25)
  point P2 (5.4535, -25)
  dimension "d19" = 0
  dimension "d20" = 0
  constraints: 8 end point, 2 parallel, 1 horizontal, 1 perpendicular
  measures "d19" distance from line of point (15.453, 25) L0
  measures "d20" distance from line of point (5.453, -25) L2
emboss "Emboss4" sketch "NamePlate" operation add depth 0.75 direction (1, 0, 0) wrap yes faces at (32.9673, 14.6667, 37.592)
emboss "Emboss5" sketch "Text" operation add depth 0.5 direction (1, 0, 0) wrap yes faces at (46.7536, 8.7868, 19.7399) contours L35 L36 L37 L38 L39 L40 L41 S6 S7 L42 S4 L12 | L12 S4 S5 L35 | L123 L124 S44 L125 L126 S45 L127 L128 S46 L12 L134 L135 S52 L136 L137 L138 L139 L11 | L11 L139 L140 L12 L155 L156 L153 L150 L151 L152 L121 L122 S42 S43 L123 | S55 L147 L148 S56 S57 L149 L150 L12 L153 L154 L155 L140 L141 L11 | L11 L141 L142 L143 S53 L12 L144 L145 L146 S55 | L22 L23 S1 S2 L24 L25 L26 L27 L12 L28 L29 L30 L31 L32 | L12 L32 L33 S3 L34 L28 L27 L13 L14 L15 L16 L17 S0 L18 L19 L20 L21 L22 | L289 S93 L290 S94 S95 L291 S96 L292 L293 L294 S97 L295 L296 L297 S98 S99 L298 L299 S100 L300 S101 S102 S103 L301 L302 L303 L12 L309 L310 L311 L312 L307 | L12 L307 S108 S109 L308 L309 L303 L304 S104 L305 S105 S106 S107 L306 L288 L289 | S53 S54 L144 L12 | L12 S46 S47 L129 S48 S49 L130 S50 L131 L132 L133 S51 L134 | L65 L66 S11 L67 S12 S13 S14 L68 L58 L59 L12 L69 S15 S16 L70 L71 | L12 L71 S17 L72 L73 L69 L59 L60 S8 L61 S9 L62 S10 L63 L64 L65 | L266 L267 L268 L269 L270 L271 L12 | L12 L271 L272 L273 L274 L275 L280 L281 L282 L283 L284 L285 S88 L286 S89 S90 S91 S92 L287 L265 L266 | L91 L92 L93 L94 L95 L96 L12 | L12 L96 L97 L98 L99 L100 L104 L105 L106 S30 L107 L112 L113 L114 L115 L116 L117 S33 S34 S35 S36 L118 L119 S37 S38 S39 S40 S41 L120 L90 L91 | L188 L189 L190 L191 L192 L193 S61 L194 S62 S63 S64 S65 L195 L173 L174 L12 L179 L180 L181 L182 L183 | L12 L183 L184 L185 S59 S60 L186 L187 L188 | L275 L276 L277 S86 S87 L278 L279 L280 L12 | L100 L101 L102 S28 S29 L103 L104 L12 | L12 L174 L175 L176 L177 L178 L179 | L81 L82 S21 L83 S22 S23 S24 L84 L74 L75 L12 L85 S25 S26 L86 L87 | L12 L87 S27 L88 L89 L85 L75 L76 S18 L77 S19 L78 S20 L79 L80 L81 | L258 L259 L260 L253 L254 L255 L12 | L12 L255 L256 S82 S83 S84 S85 L257 L258 | L107 L108 L109 S31 S32 L110 L111 L112 L12 | L203 L204 S70 L205 L196 L12 L209 L206 L207 L208 | L12 L208 L209 L196 L197 L198 L199 L200 S66 S67 S68 S69 L201 L202 L203 | L246 L233 S78 L234 S79 L235 S80 L236 L237 L238 L12 L250 S81 L251 L252 L247 | L12 L247 L248 L249 L250 L238 L239 L240 L241 L242 L243 L244 L245 L246 | L225 L226 L227 L228 L229 L230 S73 L231 S74 S75 S76 S77 L232 L210 L211 L12 L216 L217 L218 L219 L220 | L12 L220 L221 L222 S71 S72 L223 L224 L225 | L211 L212 L213 L214 L215 L216 L12 | L157 L158 L159 L160 L161 L162 S58 L163 | L261 L262 L263 L264
emboss "Emboss6" sketch "Text" operation add depth 0.4 direction (1, 0, 0) wrap yes faces at (46.6059, 14.2094, -20.0861) contours A0 | A1 | A2 | A3
fillet "Rivots" radius 0.35 4 edges at (45.4209, 14.3285, 23.5216) (45.4209, 5.8285, 23.5216) (45.4209, 14.3285, -23.5216) (45.4209, 5.8285, -23.5216)
pattern_circular "Circular Pattern1" count 2 over 360 about axis through (0, -10, 0) along (0, 1, 0) of "Emboss4"
pattern_circular "Circular Pattern2" count 2 over 360 about axis through (0, -10, 0) along (0, 1, 0) of "Emboss5"
pattern_circular "Circular Pattern3" count 2 over 360 about axis through (0, -10, 0) along (0, 1, 0) of "Emboss6"
body "Solid1"
